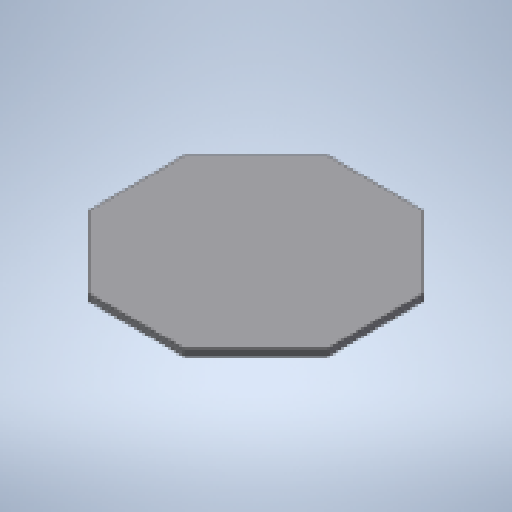
# Autodesk Inventor part: 上板
Saved by Autodesk Inventor 2025.2 (Build 292293000, 293)
## iProperties
Created: 2026-03-19
Part Number: 上板
Material: 常规
Document SubType Name: Modeling
Designer: BO‘S_SLAVE
Density: 1 g/cm^3
Appearance: 默认
Author: BO‘S_SLAVE
Autodesk Inventor part; units mm, degrees
ref_plane "YZ Plane" through (0, 0, 0) normal (1, 0, 0) x (0, 1, 0)
ref_plane "XZ Plane" through (0, 0, 0) normal (0, 1, 0) x (-1, 0, 0)
ref_plane "XY Plane" through (0, 0, 0) normal (0, 0, 1) x (1, 0, 0)
sketch "草图1" plane through (0, 0, 0) normal (0, 1, 0) x (-1, 0, 0)
  line L0 (24.7487, 24.7487) -> (-24.7487, 24.7487)
  line L1 (-24.7487, 24.7487) -> (-24.7487, -24.7487)
  line L2 (-24.7487, -24.7487) -> (24.7487, -24.7487)
  line L3 (24.7487, -24.7487) -> (24.7487, 24.7487)
  line L4 (24.7487, 24.7487) -> (-24.7487, -24.7487)
  line L5 (24.7487, -24.7487) -> (-24.7487, 24.7487)
  line L6 (-14.1421, 35.3553) -> (-35.3553, 14.1421)
  line L7 (-35.3553, -14.1421) -> (-14.1421, -35.3553)
  line L8 (14.1421, -35.3553) -> (35.3553, -14.1421)
  line L9 (35.3553, 14.1421) -> (14.1421, 35.3553)
  line L10 (14.1421, 35.3553) -> (-14.1421, 35.3553)
  line L11 (35.3553, 14.1421) -> (35.3553, -14.1421)
  line L12 (14.1421, -35.3553) -> (-14.1421, -35.3553)
  line L13 (-35.3553, -14.1421) -> (-35.3553, 14.1421)
  point P0 (0, 0)
  point P1 (0, 0)
  point P2 (-24.7487, -24.7487)
  point P3 (24.7487, -24.7487)
  point P4 (24.7487, 24.7487)
  dimension "d0" = 70
  dimension "d1" = 30
  dimension "d2" = 45
  dimension "d5" = 360
  constraints: 28 end point, 6 perpendicular, 2 midpoint, 2 parallel, 1 coincident, 1 horizontal, 17 other
  measures "d0" distance of L2.end L0.end
  measures "d1" distance of L6.start L6.end
  measures "d2" angle of L6 L1
extrude "拉伸1" add sketch "草图1" along normal blind 2
